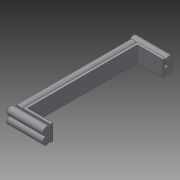
# Autodesk Inventor part: Part4
Saved by Autodesk Inventor 2015 (Build 190159000, 159)
## iProperties
Created: 2016-01-23
Part Number: Part4
Material: Generic
Document SubType Name: Modeling
Designer: sethbattis
Density: 1 g/cm^3
Appearance: Default
Author: sethbattis
Autodesk Inventor part; units mm, degrees
ref_plane "YZ Plane" through (0, 0, 0) normal (1, 0, 0) x (0, 1, 0)
ref_plane "XZ Plane" through (0, 0, 0) normal (0, 1, 0) x (-1, 0, 0)
ref_plane "XY Plane" through (0, 0, 0) normal (0, 0, 1) x (1, 0, 0)
sketch "Sketch1" plane through (0, 0, 0) normal (0, 1, 0) x (-1, 0, 0)
  line L0 (101.6, 438.15) -> (101.6, -438.15)
  line L1 (101.6, -438.15) -> (-101.6, -438.15)
  line L2 (101.6, 438.15) -> (-101.6, 438.15)
  line L3 (-101.6, -438.15) -> (-101.6, -457.2)
  line L4 (-101.6, -457.2) -> (120.65, -457.2)
  line L5 (120.65, -457.2) -> (120.65, 457.2)
  line L6 (120.65, 457.2) -> (-101.6, 457.2)
  line L7 (-101.6, 457.2) -> (-101.6, 438.15)
  line L8 (0, -640.08) -> (0, 640.08) construction
  line L9 (165.1, 0) -> (-146.05, 0) construction
  point P0 (0, 0)
  dimension "d0" = 876.3
  dimension "d1" = 203.2
  dimension "d2" = 19.05
  dimension "d3" = 19.05
  constraints: 16 end point, 5 perpendicular, 2 equal length, 2 vertical, 1 horizontal, 1 point on line, 2 other
  measures "d0" distance of L0.start L0.end
  measures "d1" distance of L0.end L1.end
  measures "d2" distance of L1.end L3.end
  measures "d3" distance between parallel lines of L0 L5
extrude "Extrusion1" add sketch "Sketch1" along normal blind 127
sketch "Sketch2" plane through (101.6, 0, 457.2) normal (1, 0, 0) x (0, 0, -1)
  circle A0 centre (-31.75, 95.25) radius 31.75
  circle A1 centre (-31.75, 31.75) radius 31.75
  line L0 (0, 0) -> (0, 127) projected
  line L1 (19.05, 127) -> (895.35, 127) projected
  point P0 (457.2, 0)
  dimension "d6" = 63.5
  constraints: 4 tangent, 2 centre point, 1 equal radius
  measures "d6" diameter of A0
extrude "Extrusion2" add sketch "Sketch2" against normal blind 285.75 contours A0 | A1
mirror "Mirror1" about plane through (0, 0, 0) normal (0, 0, 1) of "Extrusion2"
sketch "Sketch3" plane through (-120.65, 127, 457.2) normal (0, 0, 1) x (1, 0, 0)
  circle A0 centre (-31.75, -31.75) radius 31.75
  circle A1 centre (-31.75, -95.25) radius 31.75
  line L0 (0, -31.75) -> (0, 0) projected
  line L1 (0, -95.25) -> (0, -31.75) projected
  line L2 (0, 0) -> (222.25, 0) projected
  line L3 (0, -127) -> (222.25, -127) projected
  line L4 (0, -127) -> (0, -95.25) projected
  point P0 (120.65, -127)
  dimension "d9" = 63.5
  constraints: 4 tangent, 2 centre point, 1 equal radius
  measures "d9" diameter of A0
extrude "Extrusion3" add sketch "Sketch3" along normal up to surface (914.4 mm away) from surface at -914.4 contours A0 | A1
body "Solid1"
